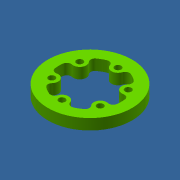
# Autodesk Inventor part: GripperMountPlate
Saved by Autodesk Inventor 2016 (Build 200138000, 138)
## iProperties
Created: 2015-09-10
Part Number: GripperMountPlate
Material: ABS-Kunststoff
Document SubType Name: Modeling
Designer: 4ndreas
Density: 1.06 g/cm^3
Appearance: Glatt - grün
Mass: 3.40696 g
Surface Area: 27.2479 cm^2
Volume: 3.21411 cm^3
Author: 4ndreas
Autodesk Inventor part; units mm, degrees
ref_plane "YZ Plane" through (0, 0, 0) normal (1, 0, 0) x (0, 1, 0)
ref_plane "XZ Plane" through (0, 0, 0) normal (0, 1, 0) x (-1, 0, 0)
ref_plane "XY Plane" through (0, 0, 0) normal (0, 0, 1) x (1, 0, 0)
sketch "Skizze1" plane through (0, 0, 0) normal (0, 0, 1) x (1, 0, 0)
  circle A0 centre (-11.2583, 6.5) radius 1.5 projected
  circle A1 centre (-11.2583, -6.5) radius 1.5 projected
  circle A2 centre (0, -13) radius 1.5 projected
  circle A3 centre (11.2583, -6.5) radius 1.5 projected
  circle A4 centre (11.2583, 6.5) radius 1.5 projected
  circle A5 centre (0, 13) radius 1.5 projected
  arc A6 (14.3761, 1.8914) -> (11.9393, 3.5783) centre (12.3932, 1.6305) ccw projected
  arc A7 (14.3761, -1.8914) -> (14.3761, 1.8914) centre (0, 0) ccw projected
  arc A8 (11.9393, -3.5783) -> (14.3761, -1.8914) centre (12.3932, -1.6305) ccw projected
  arc A9 (11.9393, -3.5783) -> (9.0685, -8.5505) centre (11.2583, -6.5) ccw projected
  arc A10 (8.826, -11.5044) -> (9.0685, -8.5505) centre (7.6087, -9.9176) ccw projected
  arc A11 (5.5501, -13.3958) -> (8.826, -11.5044) centre (0, 0) ccw projected
  arc A12 (2.8707, -12.1288) -> (5.5501, -13.3958) centre (4.7846, -11.5481) ccw projected
  arc A13 (2.8707, -12.1288) -> (-2.8707, -12.1288) centre (0, -13) ccw projected
  arc A14 (-5.5501, -13.3958) -> (-2.8707, -12.1288) centre (-4.7846, -11.5481) ccw projected
  arc A15 (-8.826, -11.5044) -> (-5.5501, -13.3958) centre (0, 0) ccw projected
  arc A16 (-9.0685, -8.5505) -> (-8.826, -11.5044) centre (-7.6087, -9.9176) ccw projected
  arc A17 (-9.0685, -8.5505) -> (-11.9393, -3.5783) centre (-11.2583, -6.5) ccw projected
  arc A18 (-14.3761, -1.8914) -> (-11.9393, -3.5783) centre (-12.3932, -1.6305) ccw projected
  arc A19 (-14.3761, 1.8914) -> (-14.3761, -1.8914) centre (0, 0) ccw projected
  arc A20 (-11.9393, 3.5783) -> (-14.3761, 1.8914) centre (-12.3932, 1.6305) ccw projected
  arc A21 (-11.9393, 3.5783) -> (-9.0685, 8.5505) centre (-11.2583, 6.5) ccw projected
  arc A22 (-8.826, 11.5044) -> (-9.0685, 8.5505) centre (-7.6087, 9.9176) ccw projected
  arc A23 (-5.5501, 13.3958) -> (-8.826, 11.5044) centre (0, 0) ccw projected
  arc A24 (-2.8707, 12.1288) -> (-5.5501, 13.3958) centre (-4.7846, 11.5481) ccw projected
  arc A25 (-2.8707, 12.1288) -> (2.8707, 12.1288) centre (0, 13) ccw projected
  arc A26 (5.5501, 13.3958) -> (2.8707, 12.1288) centre (4.7846, 11.5481) ccw projected
  arc A27 (8.826, 11.5044) -> (5.5501, 13.3958) centre (0, 0) ccw projected
  arc A28 (9.0685, 8.5505) -> (8.826, 11.5044) centre (7.6087, 9.9176) ccw projected
  arc A29 (9.0685, 8.5505) -> (11.9393, 3.5783) centre (11.2583, 6.5) ccw projected
  circle A30 centre (0, 0) radius 17.5 projected
  circle A31 centre (0, 0) radius 19.5
  point P0 (0, 0)
  dimension "d0" = 39
  constraints: 1 centre point, 1 coincident
  measures "d0" diameter of A31
extrude "Extrusion1" add sketch "Skizze1" along normal blind 5 contours A30 | A31
